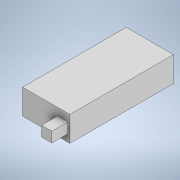
# Autodesk Inventor part: Printer power brick
Saved by Autodesk Inventor 2022 (Build 260153000, 153)
## iProperties
Created: 2021-12-03
Part Number: Printer power brick
Material: Generic
Document SubType Name: Modeling
Designer: efred
Density: 1 g/cm^3
Appearance: Default
Author: efred
Autodesk Inventor part; units mm, degrees
ref_plane "YZ Plane" through (0, 0, 0) normal (1, 0, 0) x (0, 1, 0)
ref_plane "XZ Plane" through (0, 0, 0) normal (0, 1, 0) x (-1, 0, 0)
ref_plane "XY Plane" through (0, 0, 0) normal (0, 0, 1) x (1, 0, 0)
sketch "Sketch1" plane through (0, 0, 0) normal (0, 1, 0) x (-1, 0, 0)
  line L0 (-29.5, 64.75) -> (29.5, 64.75)
  line L1 (29.5, 64.75) -> (29.5, -64.75)
  line L2 (29.5, -64.75) -> (-29.5, -64.75)
  line L3 (-29.5, -64.75) -> (-29.5, 64.75)
  line L4 (-29.5, 64.75) -> (29.5, -64.75) construction
  line L5 (29.5, 64.75) -> (-29.5, -64.75) construction
  point P0 (0, 0)
  dimension "d0" = 129.5
  dimension "d1" = 59
  constraints: 12 end point, 2 midpoint, 2 parallel, 1 horizontal, 1 perpendicular
  measures "d0" distance of L0.end L1.end
  measures "d1" distance of L1.end L2.end
extrude "Extrusion1" add sketch "Sketch1" along normal blind 31.35
sketch "Sketch2" plane through (-29.5, 0, 64.75) normal (0, 0, 1) x (1, 0, 0)
  line L0 (43.8, 22.075) -> (56.6, 22.075)
  line L1 (56.6, 22.075) -> (56.6, 9.275)
  line L2 (56.6, 9.275) -> (43.8, 9.275)
  line L3 (43.8, 9.275) -> (43.8, 22.075)
  line L4 (59, 0) -> (59, 31.35) projected
  point P0 (29.5, 0)
  point P1 (56.6, 15.675)
  point P2 (59, 15.675)
  dimension "d4" = 15.2
  dimension "d5" = 12.8
  dimension "d6" = 12.8
  constraints: 8 end point, 2 midpoint, 2 parallel, 1 horizontal, 1 horizontal alignment, 1 perpendicular
  measures "d4" distance between parallel lines of L4 L3
  measures "d5" distance between parallel lines of L3 L1
  measures "d6" distance of L0.end L1.end
extrude "Extrusion2" add sketch "Sketch2" along normal blind 20.1
body "Solid1"
